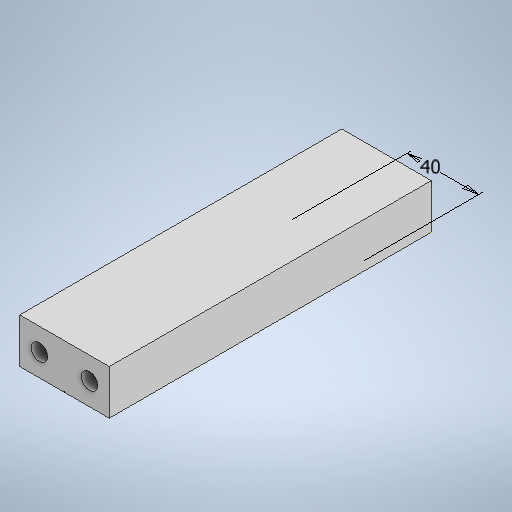
# Autodesk Inventor part: 13042026-05
Saved by Autodesk Inventor 2025.2 (Build 292293000, 293)
## iProperties
Created: 2026-05-05
Part Number: 13042026-05
Material: Generic
Document SubType Name: Modeling
Designer: Oski
Density: 1 g/cm^3
Appearance: Default
Author: Oski
Autodesk Inventor part; units mm, degrees
ref_plane "YZ Plane" through (0, 0, 0) normal (1, 0, 0) x (0, 1, 0)
ref_plane "XZ Plane" through (0, 0, 0) normal (0, 1, 0) x (-1, 0, 0)
ref_plane "XY Plane" through (0, 0, 0) normal (0, 0, 1) x (1, 0, 0)
sketch "Sketch2" plane through (0, 0, 0) normal (0, 0, 1) x (1, 0, 0)
  line L0 (-25, 12.5) -> (25, 12.5)
  line L1 (25, 12.5) -> (25, -12.5)
  line L2 (25, -12.5) -> (-25, -12.5)
  line L3 (-25, -12.5) -> (-25, 12.5)
  line L4 (-25, 12.5) -> (25, -12.5) construction
  line L5 (25, 12.5) -> (-25, -12.5) construction
  point P0 (0, 0)
  dimension "d4" = 25
  dimension "d5" = 50
  constraints: 12 end point, 2 midpoint, 2 parallel, 1 horizontal, 1 perpendicular
  measures "d4" distance of L0.end L1.end
  measures "d5" distance of L1.end L2.end
extrude "Extrusion1" add sketch "Sketch2" along normal mid plane 180
sketch "Sketch5" plane through (0, 0, -90) normal (0, 0, -1) x (-1, 0, 0)
  line L0 (-14, 0) -> (-25, 0) construction
  line L1 (-25, -12.5) -> (-25, 12.5) projected
  line L2 (14, 0) -> (25, 0) construction
  line L3 (25, 12.5) -> (25, -12.5) projected
  line L4 (-25, 0) -> (25, 0) construction
  point P0 (0, 0)
  dimension "d14" = 28
  constraints: 6 end point, 2 midpoint, 2 point on line, 1 collinear, 1 horizontal
  measures "d14" distance of L0.start L2.start
hole "Hole1" at (-14, 0, -90) direction (0, 0, 1) diameter 9.2 end through all
hole "Hole2" at (14, 0, -90) direction (0, 0, 1) diameter 9.2 end through all
sketch "Sketch6" plane through (-25, -12.5, -90) normal (0, -1, 0) x (1, 0, 0)
  point P0 (25, 90)
sketch "Sketch7" plane through (-25, -12.5, 90) normal (0, -1, 0) x (1, 0, 0)
  line L0 (45, -33.2494) -> (5, -33.2494)
  line L1 (5, -33.2494) -> (5, -146.7506)
  line L2 (5, -146.7506) -> (45, -146.7506)
  line L3 (45, -146.7506) -> (45, -33.2494)
  line L4 (45, -33.2494) -> (5, -146.7506) construction
  line L5 (5, -33.2494) -> (45, -146.7506) construction
  line L6 (25, -146.7506) -> (25, -180)
  line L7 (50, -180) -> (0, -180) projected
  line L8 (25, -33.2494) -> (25, 0)
  point P0 (25, -90)
  dimension "d29" = 40
  constraints: 16 end point, 5 midpoint, 2 parallel, 1 horizontal, 1 perpendicular, 1 point on line
  measures "d29" distance of L1.end L2.end
body "Solid1"
